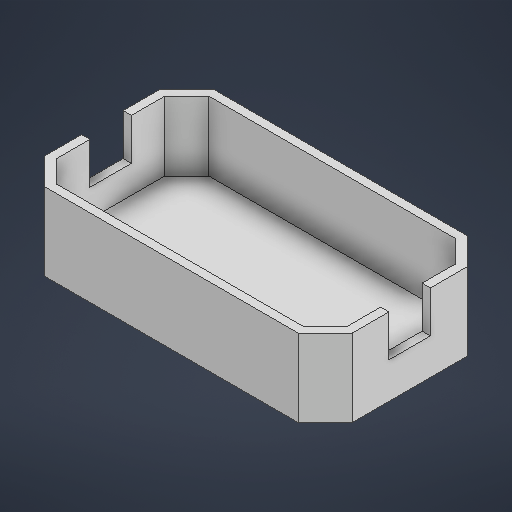
# Autodesk Inventor part: case_v1
Saved by Autodesk Inventor 2026.2 (Build 302298010, 298A)
## iProperties
Created: 2026-08-07
Part Number: case_v1
Material: Generic
Document SubType Name: Modeling
Designer: Kugelblitz
Density: 1 g/cm^3
Appearance: Default
Author: Kugelblitz
Autodesk Inventor part; units mm, degrees
ref_plane "YZ Plane" through (0, 0, 0) normal (1, 0, 0) x (0, 1, 0)
ref_plane "XZ Plane" through (0, 0, 0) normal (0, 1, 0) x (-1, 0, 0)
ref_plane "XY Plane" through (0, 0, 0) normal (0, 0, 1) x (1, 0, 0)
sketch "Sketch1" plane through (0, 0, 0) normal (0, 1, 0) x (-1, 0, 0)
  line L0 (-52.5, 27.5) -> (52.5, 27.5)
  line L1 (52.5, 27.5) -> (52.5, -27.5)
  line L2 (52.5, -27.5) -> (-52.5, -27.5)
  line L3 (-52.5, -27.5) -> (-52.5, 27.5)
  line L4 (-52.5, 27.5) -> (52.5, -27.5) construction
  line L5 (52.5, 27.5) -> (-52.5, -27.5) construction
  line L6 (52.5, 19.5) -> (44.5, 27.5)
  line L7 (52.5, -19.5) -> (44.5, -27.5)
  line L8 (-44.5, 27.5) -> (-52.5, 19.5)
  line L9 (-52.5, -19.5) -> (-44.5, -27.5)
  point P0 (0, 0)
  dimension "d0" = 105
  dimension "d1" = 55
  dimension "d4" = 45
  dimension "d5" = 8
  dimension "d6" = 8
  dimension "d7" = 8
  dimension "d8" = 8
  constraints: 20 end point, 8 point on line, 4 perpendicular, 2 midpoint, 2 parallel, 1 horizontal
  measures "d0" distance of L1.end L2.end
  measures "d1" distance of L0.end L1.end
  measures "d4" angle of L1 L6
  measures "d5" distance of L6.start L0.end
  measures "d6" distance of L1.end L7.start
  measures "d7" distance of L8.end L0.start
  measures "d8" distance of L2.end L9.start
extrude "Extrusion1" add sketch "Sketch1" along normal blind 25 contours L0 L6 L1 L7 L2 L9 L3 L8
shell "Shell1" thickness 3 outward yes removed faces 1 at (-14.8333, 25, -9.1667)
sketch "Sketch2" plane through (0, 25, 0) normal (0, 1, 0) x (1, 0, 0)
  line L0 (-55.5, 20.7426) -> (-55.5, -20.7426) projected
  line L1 (-52.5, -19.5) -> (-52.5, 19.5) projected
  line L2 (-55.5, 7.5) -> (-52.5, 7.5)
  line L3 (-52.5, 7.5) -> (-52.5, -7.5)
  line L4 (-52.5, -7.5) -> (-55.5, -7.5)
  line L5 (-55.5, -7.5) -> (-55.5, 7.5)
  line L6 (55.5, -20.7426) -> (55.5, 20.7426) projected
  line L7 (52.5, 7.5) -> (55.5, 7.5)
  line L8 (55.5, 7.5) -> (55.5, -7.5)
  line L9 (55.5, -7.5) -> (52.5, -7.5)
  line L10 (52.5, -7.5) -> (52.5, 7.5)
  line L11 (52.5, 19.5) -> (52.5, -19.5) projected
  point P0 (0, 0)
  point P1 (-54, -7.5)
  point P2 (-52.5, 0)
  point P3 (-52.5, 0)
  point P4 (54, -7.5)
  point P5 (54, 7.5)
  point P6 (52.5, 0)
  point P7 (52.5, 0)
  dimension "d10" = 15
  dimension "d11" = 0
  dimension "d12" = 0
  dimension "d13" = 15
  dimension "d14" = 0
  constraints: 16 end point, 7 midpoint, 4 parallel, 3 point on line, 2 horizontal, 2 perpendicular
  measures "d10" distance from line of point (-54, -7.5) L2
  measures "d11" distance of point (-52.5, 0) point (-52.5, 0)
  measures "d12" distance between parallel lines of L11 L10
  measures "d13" distance of point (54, -7.5) point (54, 7.5)
  measures "d14" distance of point (52.5, 0) point (52.5, 0)
extrude "Extrusion2" cut sketch "Sketch2" against normal blind 15
body "Solid1"
